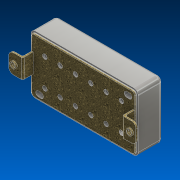
# Autodesk Inventor part: capacitor
Saved by Autodesk Inventor 2016 (Build 200138000, 138)
## iProperties
Created: 2018-12-07
Part Number: capacitor
Material: Titanium
Document SubType Name: Modeling
Designer: lesly
Density: 4.51 g/cm^3
Appearance: Chrome - Satin 1
Author: lesly
Autodesk Inventor part; units mm, degrees
ref_plane "YZ Plane" through (0, 0, 0) normal (1, 0, 0) x (0, 1, 0)
ref_plane "XZ Plane" through (0, 0, 0) normal (0, 1, 0) x (-1, 0, 0)
ref_plane "XY Plane" through (0, 0, 0) normal (0, 0, 1) x (1, 0, 0)
sketch "Sketch1" plane through (0, 0, 0) normal (0, 1, 0) x (-1, 0, 0)
  line L0 (8.0772, 17.7093) -> (-61.9228, 17.7093)
  line L1 (-61.9228, 17.7093) -> (-61.9228, -20.2907)
  line L2 (-61.9228, -20.2907) -> (8.0772, -20.2907)
  line L3 (8.0772, -20.2907) -> (8.0772, 17.7093)
  point P0 (0, 0)
  dimension "d0" = 70
  dimension "d1" = 38
  constraints: 8 end point, 2 parallel, 1 horizontal, 1 perpendicular
  measures "d0" distance of L2.end L1.end
  measures "d1" distance of L1.end L0.end
extrude "Extrusion1" add sketch "Sketch1" along normal mid plane 16
fillet "Fillet1" radius 2 4 edges at (26.9228, 8, 17.7093) (-8.0772, 8, -1.2907) (26.9228, 8, -20.2907) (61.9228, 8, -1.2907)
fillet "Fillet2" radius 3 2 edges at (61.9228, -1, 17.7093) (61.3371, 7.4142, 17.1235)
fillet "Fillet3" radius 3 2 edges at (61.3371, 7.4142, -19.7049) (61.9228, -1, -20.2907)
fillet "Fillet4" radius 3 2 edges at (-7.4914, 7.4142, 17.1235) (-8.0772, -1, 17.7093)
fillet "Fillet5" radius 3 2 edges at (-7.4914, 7.4142, -19.7049) (-8.0772, -1, -20.2907)
sketch "Sketch2" plane through (0, -8, 0) normal (0, -1, 0) x (1, 0, 0)
  arc A0 (58.9228, -20.2907) -> (61.9228, -17.2907) centre (58.9228, -17.2907) ccw
  line L0 (-7.0772, -17.2907) -> (-7.0772, 14.7093)
  arc A1 (-5.0772, 16.7093) -> (-7.0772, 14.7093) centre (-5.0772, 14.7093) ccw
  arc A2 (60.9228, 14.7093) -> (58.9228, 16.7093) centre (58.9228, 14.7093) ccw
  line L1 (60.9228, 14.7093) -> (60.9228, -17.2907)
  arc A3 (58.9228, -19.2907) -> (60.9228, -17.2907) centre (58.9228, -17.2907) ccw
  arc A4 (-7.0772, -17.2907) -> (-5.0772, -19.2907) centre (-5.0772, -17.2907) ccw
  line L2 (-1.0772, -19.2907) -> (-1.0772, -20.2907)
  line L3 (-1.0772, 16.7093) -> (-1.0772, 17.7093)
  line L4 (54.9236, -19.2907) -> (54.9236, -20.2907)
  line L5 (58.9228, -19.2907) -> (54.9236, -19.2907)
  line L6 (-1.0772, -19.2907) -> (-5.0772, -19.2907)
  line L7 (-5.0772, 16.7093) -> (-1.0772, 16.7093)
  line L8 (54.9236, 16.7093) -> (58.9228, 16.7093)
  line L9 (54.9236, -20.2907) -> (54.9236, -19.2907)
  line L10 (54.9236, 16.7093) -> (54.9236, 17.7093)
  line L11 (-1.0772, -20.2907) -> (54.9236, -20.2907)
  line L12 (-1.0772, 16.7093) -> (54.9236, 16.7093)
  line L13 (-1.0772, -19.2907) -> (54.9236, -19.2907)
  line L14 (-5.0772, -18.2907) -> (58.9228, -18.2907) projected
  point P0 (0, 0)
  point P1 (-8.0772, 14.7093)
  point P2 (58.9228, 17.7093)
  constraints: 28 end point, 10 point on circle, 6 parallel, 5 centre point, 4 perpendicular, 1 collinear, 1 point on line
extrude "Extrusion2" add sketch "Sketch2" along normal blind 1 contours L0 A1 L7 L12 L8 A2 L1 A3 L5 L13 L6 A4
fillet "Fillet6" radius 0.5 8 edges at (-6.4914, -9, 16.1235) (-7.0772, -9, -1.2907) (-6.4914, -9, -18.7049) (26.9228, -9, -19.2907) (60.3371, -9, -18.7049) (60.9228, -9, -1.2907) (60.3371, -9, 16.1235) (26.9228, -9, 16.7093)
sketch "Sketch3" plane through (0, 0, 0) normal (0, 0, 1) x (1, 0, 0)
  line L0 (60.4228, -9) -> (58.9228, -9) projected
  line L1 (60.4228, -9) -> (60.4228, -14)
  line L2 (60.4228, -9) -> (59.4228, -9)
  line L3 (59.4228, -9) -> (59.4228, -15)
  line L4 (60.4228, -16) -> (68.4228, -16)
  line L5 (68.4228, -16) -> (68.4228, -15)
  line L6 (68.4228, -15) -> (61.4228, -15)
  arc A0 (59.4228, -15) -> (60.4228, -16) centre (60.4228, -15) ccw
  arc A1 (60.4228, -14) -> (61.4228, -15) centre (61.4228, -14) ccw
  line L7 (58.9228, 8) -> (-5.0772, 8) projected
  line L8 (-6.5772, -9) -> (-5.0772, -9)
  line L9 (-6.5772, -9) -> (-6.5772, -14)
  line L10 (-6.5772, -9) -> (-5.5772, -9)
  line L11 (-5.5772, -9) -> (-5.5772, -15)
  line L12 (-6.5772, -16) -> (-14.5772, -16)
  line L13 (-14.5772, -16) -> (-14.5772, -15)
  line L14 (-14.5772, -15) -> (-7.5772, -15)
  arc A2 (-6.5772, -16) -> (-5.5772, -15) centre (-6.5772, -15) ccw
  arc A3 (-7.5772, -15) -> (-6.5772, -14) centre (-7.5772, -14) ccw
  point P0 (0, 0)
  point P1 (59.4228, -16)
  point P2 (-5.5772, -16)
  constraints: 26 end point, 8 point on circle, 6 point on line, 4 centre point, 4 tangent, 2 perpendicular, 2 vertical, 1 horizontal
extrude "Extrusion3" add sketch "Sketch3" along normal mid plane 12.5
fillet "Fillet7" radius 3 2 edges at (-14.5772, -15.5, 6.25) (-14.5772, -15.5, -6.25)
fillet "Fillet8" radius 3 2 edges at (68.4228, -15.5, 6.25) (68.4228, -15.5, -6.25)
sketch "Sketch5" plane through (0, 8, 0) normal (0, 1, 0) x (1, 0, 0)
  line L0 (-8.0772, -14.7093) -> (-8.0772, 17.2907) projected
  line L1 (61.9228, -14.7093) -> (61.9228, 17.2907) projected
  circle A0 centre (51.9228, 10.7251) radius 2.5
  circle A1 centre (41.9228, 10.7251) radius 2.5
  circle A2 centre (31.9228, 10.7251) radius 2.5
  circle A3 centre (21.9228, 10.7251) radius 2.5
  circle A4 centre (11.9228, 10.7251) radius 2.5
  circle A5 centre (1.9228, 10.7251) radius 2.5
  point P0 (0, 0)
  constraints: 6 centre point
sketch "Sketch6" plane through (-7.5772, -15, 6.25) normal (0, 1, 0) x (1, 0, 0)
  line L0 (-7, 9.5) -> (-7, 3) projected
  circle A0 centre (-3.5, 6.25) radius 1.5
  line L1 (2.5, -11.4593) -> (66.5, -11.4593) projected
  line L2 (66.5, 26.5407) -> (2.5, 26.5407) projected
  circle A1 centre (72.5, 6.25) radius 1.5
  point P0 (7.5772, 6.25)
  constraints: 2 centre point
extrude "Extrusion4" cut sketch "Sketch6" against normal blind 12.5
hole "Hole1" at (51.9228, 8, -10.7251) at (41.9228, 8, -10.7251) at (31.9228, 8, -10.7251) at (21.9228, 8, -10.7251) at (11.9228, 8, -10.7251) at (1.9228, 8, -10.7251) direction (0, -1, 0) diameter 3 depth 21 counterbore diameter 5 counterbore depth 3
sketch "Sketch7" plane through (0, -9, 0) normal (0, -1, 0) x (1, 0, 0)
  circle A0 centre (31.9228, -10.7251) radius 1.5 projected
  circle A1 centre (11.9228, -10.7251) radius 1.5 projected
  circle A2 centre (1.9228, -10.7251) radius 1.5 projected
  circle A3 centre (51.9228, -10.7251) radius 1.5 projected
  circle A4 centre (51.9228, 7.2749) radius 1.5
  circle A5 centre (1.9228, 7.2749) radius 1.5
  circle A6 centre (41.9228, -10.7251) radius 1.5 projected
  circle A7 centre (21.9228, -10.7251) radius 1.5 projected
  circle A8 centre (41.9228, 7.2749) radius 1.5
  circle A9 centre (31.9228, 7.2749) radius 1.5
  circle A10 centre (21.9228, 7.2749) radius 1.5
  circle A11 centre (11.9228, 7.2749) radius 1.5
  point P0 (0, 0)
  constraints: 6 centre point
extrude "Extrusion5" cut sketch "Sketch7" against normal blind 1 contours A4 | A5 | A8 | A9 | A10 | A11
sketch "Sketch8" plane through (0, -9, 0) normal (0, -1, 0) x (1, 0, 0)
  line L0 (58.9228, -18.7907) -> (-5.0772, -18.7907) projected
  line L1 (-0.643, -14.134) -> (-2.1755, -14.1094)
  line L2 (-2.2313, -17.5769) -> (-0.6988, -17.6015)
  arc A0 (-0.6988, -17.6015) -> (-0.643, -14.134) centre (-0.6709, -15.8678) ccw
  arc A1 (-2.1755, -14.1094) -> (-2.2313, -17.5769) centre (-2.2034, -15.8431) ccw
  line L3 (57.028, 14.4029) -> (55.4956, 14.4275)
  line L4 (55.4398, 10.96) -> (56.9723, 10.9354)
  arc A2 (56.9723, 10.9354) -> (57.028, 14.4029) centre (57.0002, 12.6692) ccw
  arc A3 (55.4956, 14.4275) -> (55.4398, 10.96) centre (55.4677, 12.6938) ccw
  point P0 (0, 0)
  point P1 (-2.321, -18.5267)
  constraints: 8 end point, 8 point on circle, 8 tangent, 4 centre point, 2 parallel
extrude "Extrusion6" cut sketch "Sketch8" against normal blind 15
sketch "Sketch9" plane through (-6.5772, -16, -6.25) normal (0, -1, 0) x (1, 0, 0)
  circle A0 centre (-4.4646, 6.25) radius 1.5004
  circle A1 centre (-4.4646, 6.25) radius 2
  line L0 (1.5, 23.9593) -> (65.5, 23.9593) projected
  line L1 (1.5, -14.0407) -> (65.5, -14.0407) projected
  circle A2 centre (71.4646, 6.25) radius 1.5004
  circle A3 centre (71.4646, 6.25) radius 2
  point P0 (6.5772, 6.25)
  dimension "d105" = 4
  constraints: 4 centre point, 2 coincident
  measures "d105" diameter of A1
extrude "Extrusion7" add sketch "Sketch9" along normal blind 1
body "Solid1"
